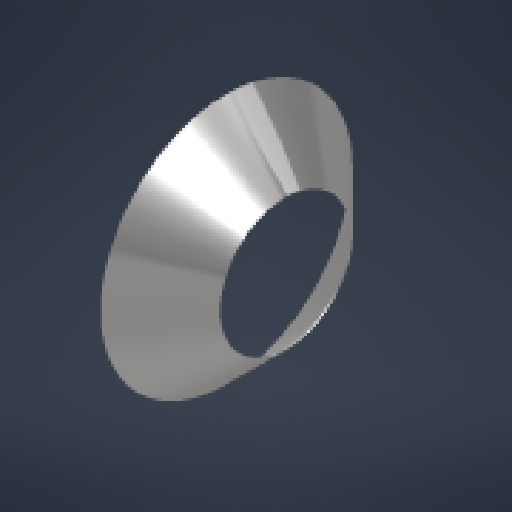
# Autodesk Inventor part: Anode
Saved by Autodesk Inventor 2025 (Build 290162000, 162)
## iProperties
Created: 2025-01-24
Part Number: Anode
Material: Сталь, легированная
Document SubType Name: Modeling
Designer: khrip
Density: 7.73 g/cm^3
Appearance: С умеренной полировкой
Author: khrip
Autodesk Inventor part; units mm, degrees
ref_plane "YZ Plane" through (0, 0, 0) normal (1, 0, 0) x (0, 1, 0)
ref_plane "XZ Plane" through (0, 0, 0) normal (0, 1, 0) x (-1, 0, 0)
ref_plane "XY Plane" through (0, 0, 0) normal (0, 0, 1) x (1, 0, 0)
sketch "Эскиз1" plane through (0, 0, 0) normal (0, 0, 1) x (1, 0, 0)
  line L0 (-7.0711, 7.0711) -> (0, 0)
  line L1 (0.1061, 0.1061) -> (-6.965, 7.1771)
  line L2 (-6.965, 7.1771) -> (-7.0711, 7.0711)
  line L3 (0, 0) -> (0.1061, 0.1061)
  line L4 (-7.7782, 7.7782) -> (-7.6721, 7.8842)
  line L5 (-7.6721, 7.8842) -> (-12.6219, 12.834)
  line L6 (-12.6219, 12.834) -> (-12.7279, 12.7279)
  line L7 (-12.7279, 12.7279) -> (-7.7782, 7.7782)
  line L8 (-15.2947, 0) -> (2.6729, 0) projected
  dimension "d0" = 7
  dimension "d1" = 1
  dimension "d2" = 0.15
  constraints: 16 end point, 2 parallel, 1 collinear, 1 perpendicular, 7 other
  measures "d0" distance of L5.end L4.end
  measures "d1" distance between parallel lines of L2 L4
  measures "d2" distance between parallel lines of L7 L5
revolve "Вращение1" add sketch "Эскиз1" angle 360 about axis through (-10, 0, 0) along (1, 0, 0) contours L7 L6 L5 L4
